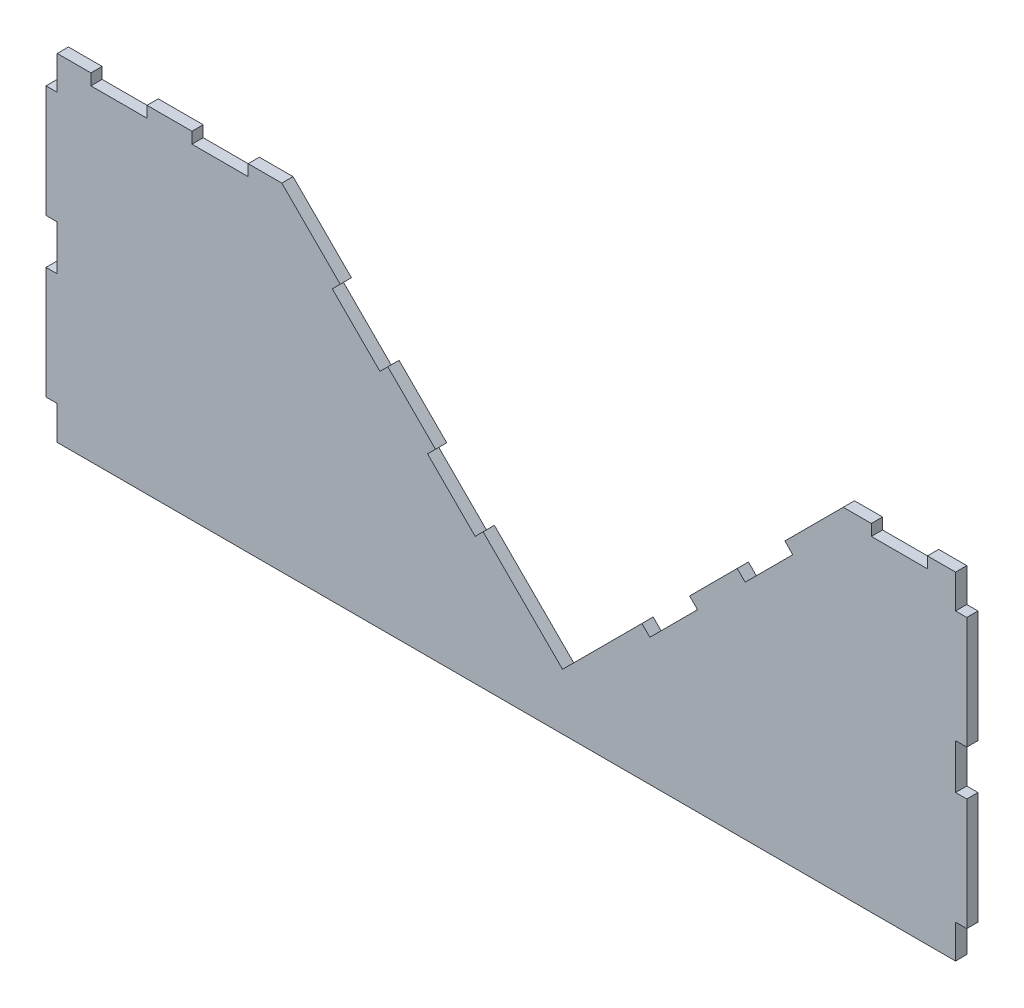
# Autodesk Inventor part: Fondo
Saved by Autodesk Inventor 2022 (Build 260153000, 153)
## iProperties
Created: 2022-06-06
Part Number: Fondo
Material: Generic
Document SubType Name: Modeling
Designer: ADMIN
Density: 1 g/cm^3
Appearance: Default
Author: ADMIN
Autodesk Inventor part; units mm, degrees
ref_plane "YZ Plane" through (0, 0, 0) normal (1, 0, 0) x (0, 1, 0)
ref_plane "XZ Plane" through (0, 0, 0) normal (0, 1, 0) x (-1, 0, 0)
ref_plane "XY Plane" through (0, 0, 0) normal (0, 0, 1) x (1, 0, 0)
sketch "Sketch1" plane through (0, 0, 0) normal (0, 0, 1) x (1, 0, 0)
  line L0 (150, -75) -> (-250, -75) projected
  line L1 (150, 75) -> (150, -75) projected
  line L2 (-250, 75) -> (-235, 75) projected
  line L3 (-250, -75) -> (-250, 75) projected
  line L4 (-255, -10) -> (-255, -60) projected
  line L5 (-255, -60) -> (-250, -60) projected
  line L6 (-250, -10) -> (-250, -60) projected
  line L7 (-255, -10) -> (-250, -10) projected
  line L8 (-255, 60) -> (-255, 10) projected
  line L9 (-255, 10) -> (-250, 10) projected
  line L10 (-250, 60) -> (-250, 10) projected
  line L11 (-255, 60) -> (-250, 60) projected
  line L12 (150, 60) -> (150, 10) projected
  line L13 (150, 10) -> (155, 10) projected
  line L14 (155, 60) -> (155, 10) projected
  line L15 (150, 60) -> (155, 60) projected
  line L16 (150, -10) -> (150, -60) projected
  line L17 (150, -60) -> (155, -60) projected
  line L18 (155, -10) -> (155, -60) projected
  line L19 (150, -10) -> (155, -10) projected
  line L20 (100, 75) -> (112.5, 75) projected
  line L21 (-25, -50) -> (10.3553, -14.6447) projected
  line L22 (-150, 75) -> (-123.9949, 48.9949) projected
  line L23 (-60.3553, -14.6447) -> (-63.8909, -18.1802) projected
  line L24 (-63.8909, -18.1802) -> (-85.1041, 3.033) projected
  line L25 (-85.1041, 3.033) -> (-81.5685, 6.5685) projected
  line L26 (-102.7817, 27.7817) -> (-81.5685, 6.5685) projected
  line L27 (-102.7817, 27.7817) -> (-106.3173, 24.2462) projected
  line L28 (-106.3173, 24.2462) -> (-127.5305, 45.4594) projected
  line L29 (-127.5305, 45.4594) -> (-123.9949, 48.9949) projected
  line L30 (73.9949, 48.9949) -> (100, 75) projected
  line L31 (73.9949, 48.9949) -> (77.5305, 45.4594) projected
  line L32 (77.5305, 45.4594) -> (56.3173, 24.2462) projected
  line L33 (56.3173, 24.2462) -> (52.7817, 27.7817) projected
  line L34 (31.5685, 6.5685) -> (52.7817, 27.7817) projected
  line L35 (31.5685, 6.5685) -> (35.1041, 3.033) projected
  line L36 (35.1041, 3.033) -> (13.8909, -18.1802) projected
  line L37 (13.8909, -18.1802) -> (10.3553, -14.6447) projected
  line L38 (-60.3553, -14.6447) -> (-25, -50) projected
  line L39 (-210, 75) -> (-210, 70) projected
  line L40 (-210, 70) -> (-235, 70) projected
  line L41 (-235, 70) -> (-235, 75) projected
  line L42 (137.5, 75) -> (150, 75) projected
  line L43 (137.5, 75) -> (137.5, 70) projected
  line L44 (137.5, 70) -> (112.5, 70) projected
  line L45 (112.5, 70) -> (112.5, 75) projected
  line L46 (-165, 75) -> (-150, 75) projected
  line L47 (-165, 75) -> (-165, 70) projected
  line L48 (-165, 70) -> (-190, 70) projected
  line L49 (-190, 70) -> (-190, 75) projected
  line L50 (-210, 75) -> (-190, 75) projected
  point P0 (0, 0)
extrude "Extrusion1" add sketch "Sketch1" along normal blind 5
sketch "Sketch2" plane through (0, 0, 5) normal (0, 0, 1) x (1, 0, 0)
  point P0 (0, 0)
body "Solid1"
